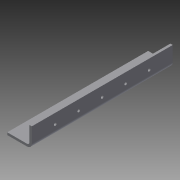
# Autodesk Inventor part: long_angle_bracket
Saved by Autodesk Inventor 2015 SP1 (Build 190203100, 203)
## iProperties
Created: 2015-11-04
Part Number: long_angle_bracket
Material: Generic
Document SubType Name: Sheet Metal
Designer: elilitwack
Density: 1 g/cm^3
Sheet Metal Rule: Default
Appearance: Default
Author: elilitwack
Autodesk Inventor part; units mm, degrees
ref_plane "YZ Plane" through (0, 0, 0) normal (1, 0, 0) x (0, 1, 0)
ref_plane "XZ Plane" through (0, 0, 0) normal (0, 1, 0) x (-1, 0, 0)
ref_plane "XY Plane" through (0, 0, 0) normal (0, 0, 1) x (1, 0, 0)
sketch "Sketch1" plane through (0, 0, 0) normal (0, 1, 0) x (-1, 0, 0)
  line L0 (0, 0) -> (25.4, 0)
  line L1 (25.4, 0) -> (25.4, -180.34)
  line L2 (25.4, -180.34) -> (0, -180.34)
  line L3 (0, -180.34) -> (0, 0)
  dimension "d0" = 25.4
  dimension "d1" = 180.34
  measures "d0" distance of L1.end L2.end
  measures "d1" distance of L0.end L1.end
extrude "Plate1" add sketch "Sketch1" along normal blind 3.048
sketch "Sketch2" plane through (3.048, 6.096, -180.34) normal (1, 0, 0) x (0, 1, 0)
  line L0 (0, 180.34) -> (0, 0)
  line L1 (0, 0) -> (19.304, 0)
  line L2 (19.304, 0) -> (19.304, 180.34)
  line L3 (19.304, 180.34) -> (0, 180.34)
  constraints: 6 end point, 1 horizontal, 1 perpendicular, 1 vertical
edge flange "Flange1" height 25.4 angle 90 thickness 3.048 bend radius 3.048 thickness toward (1, 0, 0) relief tear relief width 3.048 relief depth 1.524 edges at (0, 3.048, -90.17) wall of the first edge with corners at (3.048, 6.096, 0) (3.048, 6.096, -180.34) (3.048, 25.4, -180.34) (3.048, 25.4, 0)
bend "Bend1"
corner "Corner1"
sketch "Sketch3" plane through (0, 0, 0) normal (0, -1, 0) x (1, 0, 0)
  line L0 (-25.4, 0) -> (-25.4, -180.34) projected
  line L1 (-25.4, -180.34) -> (0, -180.34) construction
  line L2 (-12.7, -180.34) -> (-12.7, -150.2833) construction
  line L3 (-12.7, -150.2833) -> (-12.7, -120.2267) construction
  line L4 (-12.7, -120.2267) -> (-12.7, -90.17) construction
  line L5 (-12.7, -90.17) -> (-12.7, -60.1133) construction
  line L6 (-12.7, -60.1133) -> (-12.7, -30.0567) construction
  line L7 (-12.7, -30.0567) -> (-12.7, 0) construction
  line L8 (0, 0) -> (-25.4, 0) construction
  dimension "d13" = 12.7
  constraints: 12 end point, 5 coincident, 5 collinear, 5 point on line, 2 midpoint, 1 vertical
  measures "d13" distance between parallel lines of L0 L4
hole "Hole1" at (-12.7, 0, -120.2267) at (-12.7, 0, -150.2833) at (-12.7, 0, -90.17) at (-12.7, 0, -60.1133) at (-12.7, 0, -30.0567) direction (0, 1, 0) diameter 3.5719 depth 3.048 tip angle 118
sketch "Sketch4" plane through (6.096, 25.4, 0) normal (1, 0, 0) x (0, 0, -1)
  line L0 (0, -12.7) -> (30.0567, -12.7) construction
  line L1 (30.0567, -12.7) -> (60.1133, -12.7) construction
  line L2 (60.1133, -12.7) -> (90.17, -12.7) construction
  line L3 (90.17, -12.7) -> (120.2267, -12.7) construction
  line L4 (120.2267, -12.7) -> (150.2833, -12.7) construction
  line L5 (150.2833, -12.7) -> (180.34, -12.7) construction
  line L6 (180.34, -25.4) -> (0, -25.4) projected
  line L7 (180.34, 0) -> (180.34, -19.304) projected
  line L8 (0, -19.304) -> (0, 0) projected
  dimension "d21" = 12.7
  constraints: 12 end point, 7 point on line, 5 coincident, 5 collinear, 1 horizontal
  measures "d21" distance between parallel lines of L6 L2
hole "Hole2" at (6.096, 12.7, -30.0567) at (6.096, 12.7, -60.1133) at (6.096, 12.7, -90.17) at (6.096, 12.7, -120.2267) at (6.096, 12.7, -150.2833) direction (-1, 0, 0) diameter 3.5719 depth 3.048 tip angle 118
equation "\"d0\" = cb_outer_diameter"
equation "\"d1\" = bh_length"
equation "\"d13\" = 0.5 * cb_outer_diameter"
equation "\"d14\" = rv_hole_diameter"
equation "\"d19\" = Thickness"
equation "\"d21\" = 0.5 * cb_outer_diameter"
equation "\"d22\" = rv_hole_diameter"
equation "\"d27\" = Thickness"
equation "\"d3\" = BendReliefWidth"
equation "\"d4\" = BendReliefDepth"
equation "\"d5\" = MinimumRemnant"
equation "\"d6\" = BendRadius"
equation "\"d9\" = BendRadius"
equation "\"d10\" = CornerReliefSize"
equation "\"d11\" = GapSize"
equation "\"d12\" = JacobiRadiusSize"
equation "\"BendRadius\" = Thickness"
equation "\"BendReliefWidth\" = Thickness"
equation "\"BendReliefDepth\" = 0.5 * Thickness"
equation "\"CornerReliefSize\" = 4 * Thickness"
equation "\"MinimumRemnant\" = 2 * Thickness"
equation "\"TransitionRadius\" = BendRadius"
equation "\"JacobiRadiusSize\" = BendRadius"
equation "\"GapSize\" = Thickness"
equation "\"bh_width\" = 87.63"
equation "\"bh_length\" = 180.34"
equation "\"bh_height\" = 25.4"
equation "\"bh_metal_width\" = 3.048"
equation "\"cpn_diameter\" = 69.85"
equation "\"cpn_length\" = 311.15"
equation "\"cmp_foot_seperation_long\" = 139.954"
equation "\"cmp_foot_seperation_short\" = 36.068"
equation "\"cmp_mounting_margins\" = 6.35"
equation "\"cmp_foot_bolt_diameter\" = 6.35"
equation "\"spd_fillet_size\" = 3.175"
equation "\"cb_outer_diameter\" = 25.4"
equation "\"cb_wall_thickness\" = 1.5875"
equation "\"cb_length\" = 508"
equation "\"pdb_mounting_holes_short\" = 104.394"
equation "\"cb_pdb_low_mount_offset\" = 25.4"
equation "\"pdb_mounting_holes_long\" = 182.2704"
equation "\"pdb_ziptie_hole_diameter\" = 5.334"
equation "\"d2\" = BendRadius"
equation "\"rv_hole_diameter\" = 3.57187"
equation "\"Thickness\" = 3.048"
body "Solid1"
